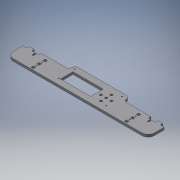
# Autodesk Inventor part: A8-0011
Saved by Autodesk Inventor 2016 SP2 (Build 200236200, 236)
## iProperties
Created: 2017-04-22
Part Number: A8-0011
Material: Generic
Document SubType Name: Modeling
Designer: EV
Density: 1 g/cm^3
Appearance: Default
Author: EV
Autodesk Inventor part; units mm, degrees
ref_plane "YZ Plane" through (0, 0, 0) normal (1, 0, 0) x (0, 1, 0)
ref_plane "XY Plane" through (0, 0, 0) normal (0, 0, 1) x (1, 0, 0)
sketch "Sketch1" plane through (0, 0, 0) normal (0, 1, 0) x (-1, 0, 0)
  line L0 (208, 0) -> (-208, 0)
  line L1 (-228, -20) -> (-228, -52)
  line L2 (-228, -52) -> (-215.25, -52)
  line L3 (-215.25, -52) -> (-215.25, -60)
  line L4 (-215.25, -60) -> (-200.25, -60)
  line L5 (-200.25, -60) -> (-200.25, -52)
  line L6 (-200.25, -52) -> (-176.75, -52)
  line L7 (-176.75, -52) -> (-176.75, -60)
  line L8 (-176.75, -60) -> (-88, -60)
  line L9 (-88, -60) -> (-88, -80)
  line L10 (-88, -80) -> (88, -80)
  line L11 (88, -80) -> (88, -60)
  line L12 (88, -60) -> (176.75, -60)
  line L13 (176.75, -60) -> (176.75, -52)
  line L14 (176.75, -52) -> (200.25, -52)
  line L15 (200.25, -52) -> (200.25, -60)
  line L16 (200.25, -60) -> (215.25, -60)
  line L17 (215.25, -60) -> (215.25, -52)
  line L18 (215.25, -52) -> (228, -52)
  line L19 (228, -52) -> (228, -20)
  line L20 (0, -80) -> (0, 0) construction
  arc A0 (228, -20) -> (208, 0) centre (208, -20) ccw
  arc A1 (-208, 0) -> (-228, -20) centre (-208, -20) ccw
  line L21 (75, -19) -> (-23, -19)
  line L22 (-23, -19) -> (-23, -60)
  line L23 (-23, -60) -> (75, -60)
  line L24 (75, -60) -> (75, -19)
  line L25 (155.25, -4) -> (147.05, -4)
  line L26 (147.05, -4) -> (147.05, -12.2)
  line L27 (147.05, -12.2) -> (155.25, -12.2)
  line L28 (155.25, -12.2) -> (155.25, -4)
  line L29 (155.25, -23) -> (147.05, -23)
  line L30 (147.05, -23) -> (147.05, -31.2)
  line L31 (147.05, -31.2) -> (155.25, -31.2)
  line L32 (155.25, -31.2) -> (155.25, -23)
  line L33 (155.25, -42) -> (147.05, -42)
  line L34 (147.05, -42) -> (147.05, -50.2)
  line L35 (147.05, -50.2) -> (155.25, -50.2)
  line L36 (155.25, -50.2) -> (155.25, -42)
  line L37 (151.15, -42) -> (151.15, -31.2) construction
  line L38 (151.15, -23) -> (151.15, -12.2) construction
  line L39 (-155.25, -4) -> (-147.05, -4)
  line L40 (-147.05, -4) -> (-147.05, -12.2)
  line L41 (-147.05, -12.2) -> (-155.25, -12.2)
  line L42 (-155.25, -12.2) -> (-155.25, -4)
  line L43 (-155.25, -23) -> (-147.05, -23)
  line L44 (-147.05, -23) -> (-147.05, -31.2)
  line L45 (-147.05, -31.2) -> (-155.25, -31.2)
  line L46 (-155.25, -31.2) -> (-155.25, -23)
  line L47 (-155.25, -42) -> (-147.05, -42)
  line L48 (-147.05, -42) -> (-147.05, -50.2)
  line L49 (-147.05, -50.2) -> (-155.25, -50.2)
  line L50 (-155.25, -50.2) -> (-155.25, -42)
  line L51 (-151.15, -42) -> (-151.15, -31.2) construction
  line L52 (-151.15, -23) -> (-151.15, -12.2) construction
  line L53 (79, -69.5) -> (-74, -69.5) construction
  line L54 (-74, -69.5) -> (-74, -18.5) construction
  line L55 (-74, -18.5) -> (79, -18.5) construction
  line L56 (79, -18.5) -> (79, -69.5) construction
  line L57 (-35.5, -40) -> (-69.5, -40) construction
  line L58 (-52.5, -57) -> (-52.5, -23) construction
  line L59 (188, -52) -> (188, -48)
  line L60 (188, -48) -> (189.25, -48)
  line L61 (189.25, -48) -> (189.25, -45)
  line L62 (189.25, -45) -> (188, -45)
  line L63 (188, -45) -> (188, -40)
  line L64 (188, -40) -> (184.5, -40)
  line L65 (184.5, -40) -> (184.5, -45)
  line L66 (184.5, -45) -> (183.25, -45)
  line L67 (183.25, -45) -> (183.25, -48)
  line L68 (183.25, -48) -> (184.5, -48)
  line L69 (184.5, -48) -> (184.5, -52)
  line L70 (-184.5, -52) -> (-184.5, -48)
  line L71 (-184.5, -48) -> (-183.25, -48)
  line L72 (-183.25, -48) -> (-183.25, -45)
  line L73 (-183.25, -45) -> (-184.5, -45)
  line L74 (-184.5, -45) -> (-184.5, -40)
  line L75 (-184.5, -40) -> (-188, -40)
  line L76 (-188, -40) -> (-188, -45)
  line L77 (-188, -45) -> (-189.25, -45)
  line L78 (-189.25, -45) -> (-189.25, -48)
  line L79 (-189.25, -48) -> (-188, -48)
  line L80 (-188, -48) -> (-188, -52)
  point P0 (228, 0)
  point P1 (-228, 0)
  point P2 (151.15, -36.6)
  point P3 (151.15, -17.6)
  point P4 (-151.15, -36.6)
  point P5 (-151.15, -17.6)
  point P6 (-52.5, -40)
  point P7 (-52.5, -40)
  dimension "d0" = 456
  dimension "d1" = 80
  dimension "d2" = 60
  dimension "d3" = 8
  dimension "d4" = 140
  dimension "d5" = 23.5
  dimension "d6" = 15
  dimension "d7" = 12.75
  dimension "d8" = 20
  dimension "d9" = 19
  dimension "d10" = 41
  dimension "d11" = 98
  dimension "d12" = 153
  dimension "d13" = 8.2
  dimension "d14" = 8.2
  dimension "d15" = 72.75
  dimension "d16" = 4
  dimension "d17" = 23
  dimension "d18" = 42
  dimension "d19" = 18.5
  dimension "d20" = 51
  dimension "d21" = 153
  dimension "d22" = 149
  dimension "d23" = 40
  dimension "d24" = 29.5
  dimension "d25" = 34
  dimension "d26" = 34
  dimension "d27" = 4
  dimension "d28" = 3
  dimension "d29" = 5
  dimension "d30" = 6
  dimension "d31" = 3.5
  dimension "d32" = 40
  dimension "d34" = 3.5
  dimension "d35" = 6
  dimension "d36" = 40
  constraints: 162 end point, 35 point on line, 32 perpendicular, 18 symmetric about line, 11 parallel, 10 coincident, 10 midpoint, 8 equal length, 6 horizontal, 5 vertical, 4 point on circle, 4 tangent, 3 collinear, 2 centre point, 1 equal radius, 6 other
  measures "d0" distance of point (228, 0) point (-228, 0)
  measures "d1" distance between parallel lines of L10 L0
  measures "d2" distance between parallel lines of L0 L12
  measures "d3" distance of L16.end L17.end
  measures "d4" distance between parallel lines of L19 L11
  measures "d5" distance between parallel lines of L13 L15
  measures "d6" distance of L15.end L16.end
  measures "d7" distance between parallel lines of L19 L17
  measures "d8" radius of A0
  measures "d9" distance between parallel lines of L0 L21
  measures "d10" distance between parallel lines of L23 L21
  measures "d11" distance of L21.start L21.end
  measures "d12" distance between parallel lines of L19 L24
  measures "d13" distance of L25.start L25.end
  measures "d14" distance of L27.end L25.start
  measures "d15" distance between parallel lines of L19 L28
  measures "d16" distance between parallel lines of L0 L25
  measures "d17" distance between parallel lines of L0 L29
  measures "d18" distance between parallel lines of L0 L33
  measures "d19" distance between parallel lines of L0 L55
  measures "d20" distance of L55.end L53.start
  measures "d21" distance of L54.end L55.end
  measures "d22" distance between parallel lines of L19 L56
  measures "d23" distance between parallel lines of L0 L57
  measures "d24" distance between parallel lines of L22 L58
  measures "d25" distance of L57.start L57.end
  measures "d26" distance of L58.start L58.end
  measures "d27" distance of L68.end L69.end
  measures "d28" distance of L66.end L67.end
  measures "d29" distance of L64.end L65.end
  measures "d30" distance between parallel lines of L67 L61
  measures "d31" distance between parallel lines of L59 L69
  measures "d32" distance between parallel lines of L19 L59
  measures "d34" distance between parallel lines of L80 L70
  measures "d35" distance between parallel lines of L72 L78
  measures "d36" distance between parallel lines of L1 L80
extrude "Extrusion1" add sketch "Sketch1" along normal blind 8 contours A0 L19 L18 L17 L16 L15 L14 L59 L60 L61 L62 L63 L64 L65 L66 L67 L68 L69 L13 L12 L11 L10 L9 L8 L7 L6 L70 L71 L72 L73 L74 L75 L76 L77 L78 L79 L80 L5 L4 L3 L2 L1 A1 L0
fillet "Fillet1" radius 10 4 edges at (-88, 4, -60) (-88, 4, -80) (88, 4, -80) (88, 4, -60)
hole "Hole1" at (-151.15, 0, -36.6) at (-151.15, 0, -17.6) at (151.15, 0, -17.6) at (151.15, 0, -36.6) at (-79, 0, -69.5) at (-79, 0, -18.5) at (74, 0, -18.5) at (74, 0, -69.5) direction (0, 1, 0) diameter 3.5 end through all
hole "Hole2" at (35.5, 0, -40) at (52.5, 0, -57) at (52.5, 0, -40) at (69.5, 0, -40) at (52.5, 0, -23) direction (0, 1, 0) diameter 8 end through all
ref_plane "Work Plane2" through (0, 4, 0) normal (0, 1, 0) x (-1, 0, 0)
equation "\"d34\" = d31"
equation "\"d35\" = d30"
equation "\"d36\" = d32"
equation "\"d55\" = 0.5 * THICKNESS"
equation "\"THICKNESS\" = 8"
body "Solid1"
